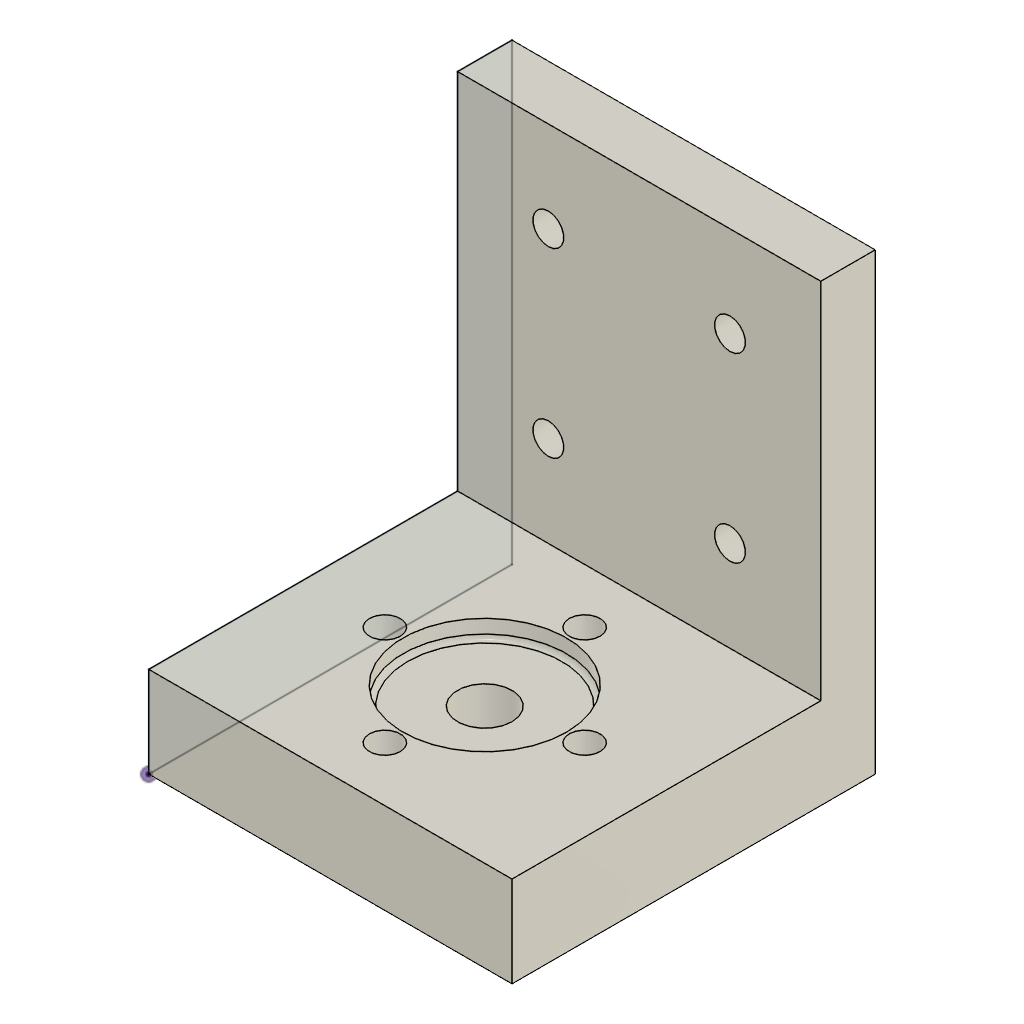
A4-1 (Autodesk Fusion 360 design; units mm, degrees)
part number: 2026-09-15-13-49-53-125
Autodesk Fusion 360 part; units mm, degrees
sketch "Sketch1" plane through (0, 0, 0) normal (1, 0, 0) x (0, 1, 0)
  line L0 (0, 0) -> (40, 0)
  line L1 (40, 0) -> (40, 50)
  line L2 (40, 50) -> (34, 50)
  line L3 (34, 50) -> (34, 10)
  line L4 (34, 10) -> (0, 10)
  line L5 (0, 10) -> (0, 0)
  dimension "d10" = 50
  dimension "d11" = 40
  dimension "d12" = 10
  dimension "d13" = 6
  constraint coincident L0.start L5.end
  constraint horizontal L0
  constraint perpendicular L0 L1
  constraint perpendicular L1 L2
  constraint perpendicular L2 L3
  constraint perpendicular L1 L4
  constraint perpendicular L0 L5
  measures "d10" distance of L0.end L1.end
  measures "d11" distance of L0.start L0.end
  measures "d12" distance of L0.start L4.end
  measures "d13" distance of L1.end L2.end
extrude "Extrude1" add sketch "Sketch1" along normal blind 40
hole "Hole1" at (30, 34, 40) direction (0, 1, 0) diameter 3.4 end through all
hole "Hole2" at (10, 34, 40) direction (0, 1, 0) diameter 3.4 end through all
hole "Hole3" at (10, 34, 20) direction (0, 1, 0) diameter 3.4 end through all
hole "Hole4" at (30, 34, 20) direction (0, 1, 0) diameter 3.4 end through all
sketch "Sketch3" plane through (0, 0, 10) normal (0, 0, 1) x (-1, 0, 0)
  line L0 (0, -34) -> (0, 0)
  line L1 (0, 0) -> (-40, 0)
  line L2 (-40, 0) -> (-40, -34)
  line L3 (-40, -34) -> (0, -34)
  circle A0 centre (-20, -17) radius 9
  line L4 (0, -34) -> (0, 0)
  dimension "d36" = 18
  dimension "d37" = 17
  dimension "d38" = 20
  measures "d36" diameter of A0
  measures "d37" distance of L1 A0.centre
  measures "d38" distance of A0.centre L4
extrude "Extrude2" cut sketch "Sketch3" against normal blind 2 contours A0
hole "Hole5" at (20, 17, 10) direction (0, 0, -1) diameter 6 end through all
fillet "Fillet1" radius 0.5 1 edges at (28.3909, 13.7455, 8)
sketch "Sketch4" plane through (0, 0, 10) normal (0, 0, 1) x (-1, 0, 0)
  circle A0 centre (-20, -17) radius 9
  line L0 (0, -34) -> (0, 0)
  line L1 (0, 0) -> (-40, 0)
  line L2 (-40, 0) -> (-40, -34)
  line L3 (-40, -34) -> (0, -34)
  circle A1 centre (-20, -28) radius 1.7
  circle A2 centre (-31, -17) radius 1.7
  circle A3 centre (-20, -6) radius 1.7
  circle A4 centre (-9, -17) radius 1.7
  dimension "d48" = 3.4
  dimension "d49" = 3.4
  dimension "d50" = 3.4
  dimension "d51" = 3.4
  measures "d48" diameter of A1
  measures "d49" diameter of A2
  measures "d50" diameter of A3
  measures "d51" diameter of A4
extrude "Extrude3" cut sketch "Sketch4" against normal through all contours A1 | A2 | A3 | A4
equation "b = 40 mm"
equation "L2 = 1.25 * b"
equation "L1 = b"
equation "H2 = 6 mm"
equation "H1 = 10 mm"
equation "d10 = L2"
equation "d11 = L1"
equation "d12 = H1"
equation "d13 = H2"
equation "d14 = b"
